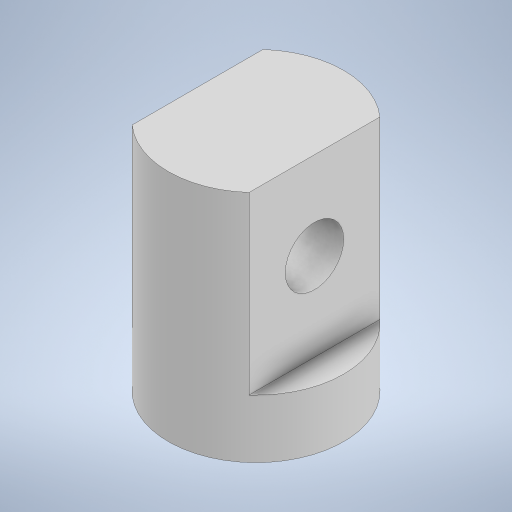
# Autodesk Inventor part: anchor_end_3.0mm_new
Saved by Autodesk Inventor 2024 (Build 280153000, 153)
## iProperties
Created: 2024-06-07
Part Number: anchor_end_3.0mm_new
Material: 일반
Document SubType Name: Modeling
Designer: Gihyeok Na
Density: 1 g/cm^3
Appearance: 기본값
Author: Gihyeok Na
Autodesk Inventor part; units mm, degrees
ref_plane "YZ Plane" through (0, 0, 0) normal (1, 0, 0) x (0, 1, 0)
ref_plane "XZ Plane" through (0, 0, 0) normal (0, 1, 0) x (-1, 0, 0)
ref_plane "XY Plane" through (0, 0, 0) normal (0, 0, 1) x (1, 0, 0)
sketch "스케치2" plane through (0, 0, 0) normal (0, 1, 0) x (-1, 0, 0)
  circle A0 centre (0, 0) radius 1.5
  circle A1 centre (0, 0) radius 0.9
  dimension "d0" = 3
  dimension "d6" = 1.8
  constraints: 2 centre point, 2 coincident
  measures "d0" diameter of A0
  measures "d6" diameter of A1
extrude "돌출1" add sketch "스케치2" along normal blind 1
sketch "스케치4" plane through (0, 1, 0) normal (0, 1, 0) x (1, 0, 0)
  line L0 (1, -3.1) -> (-1, -3.1)
  line L1 (-1, -3.1) -> (-1, 3.1)
  line L2 (-1, 3.1) -> (1, 3.1)
  line L3 (1, 3.1) -> (1, -3.1)
  line L4 (1, -3.1) -> (-1, 3.1) construction
  line L5 (-1, -3.1) -> (1, 3.1) construction
  circle A0 centre (0, 0) radius 1.5 projected
  point P0 (1, 1.118)
  point P1 (-1, 1.118)
  point P2 (-1, -1.118)
  point P3 (1, -1.118)
  dimension "d7" = 2
  constraints: 12 end point, 2 midpoint, 2 parallel, 1 horizontal, 1 perpendicular
  measures "d7" distance of L1.end L2.end
extrude "돌출5" add sketch "스케치4" along normal blind 3 contours A0 L1 L3
sketch "스케치6" plane through (1, 1, 1.118) normal (1, 0, 0) x (0, 0, -1)
  circle A0 centre (1.118, 1.5) radius 0.5
  line L0 (0, 3) -> (2.2361, 3) projected
  point P0 (1.118, -1)
  dimension "d22" = 1
  dimension "d23" = 1.5
  constraints: 1 centre point
  measures "d22" diameter of A0
  measures "d23" distance from line of L0 A0.centre
extrude "돌출6" cut sketch "스케치6" along normal through all both and the other way through all
